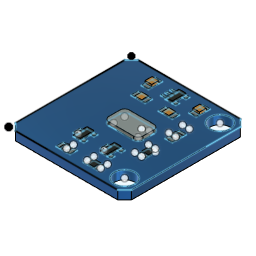
MPL3115A2 (Autodesk Fusion 360 design; units mm, degrees)
Autodesk Fusion 360 part; units mm, degrees
sketch "Esquisse1" plane through (0, 0, 0) normal (0, 0, 1) x (1, 0, 0)
  line L0 (1, 0) -> (16, 0)
  line L1 (17, 1) -> (17, 17)
  line L2 (16, 18) -> (1, 18)
  line L3 (0, 17) -> (0, 1)
  circle A0 centre (15, 16) radius 1.5
  circle A1 centre (15, 2) radius 1.5
  line L4 (10.8, 7.5) -> (7.2, 7.5)
  line L5 (6.5, 8.2) -> (6.5, 9.8)
  line L6 (7.2, 10.5) -> (10.8, 10.5)
  line L7 (11.5, 9.8) -> (11.5, 8.2)
  arc A2 (7.2, 10.5) -> (6.5, 9.8) centre (7.2, 9.8) ccw
  arc A3 (11.5, 9.8) -> (10.8, 10.5) centre (10.8, 9.8) ccw
  arc A4 (6.5, 8.2) -> (7.2, 7.5) centre (7.2, 8.2) ccw
  arc A5 (10.8, 7.5) -> (11.5, 8.2) centre (10.8, 8.2) ccw
  line L8 (14, 12) -> (13, 12)
  line L9 (13, 12) -> (13, 10)
  line L10 (13, 10) -> (14, 10)
  line L11 (14, 10) -> (14, 12)
  line L12 (14, 8) -> (13, 8)
  line L13 (13, 8) -> (13, 6)
  line L14 (13, 6) -> (14, 6)
  line L15 (14, 6) -> (14, 8)
  line L16 (12.5, 17) -> (11.5, 17)
  line L17 (11.5, 17) -> (11.5, 15)
  line L18 (11.5, 15) -> (12.5, 15)
  line L19 (12.5, 15) -> (12.5, 17)
  line L20 (12, 2) -> (10, 2)
  line L21 (10, 2) -> (10, 1)
  line L22 (10, 1) -> (12, 1)
  line L23 (12, 1) -> (12, 2)
  line L24 (8, 2) -> (6, 2)
  line L25 (6, 2) -> (6, 1)
  line L26 (6, 1) -> (8, 1)
  line L27 (8, 1) -> (8, 2)
  line L28 (10.97, 5.5) -> (10, 5.5)
  line L29 (10, 5.5) -> (10, 3.5)
  line L30 (10, 3.5) -> (10.97, 3.5)
  line L31 (10.97, 3.5) -> (10.97, 5.5)
  line L32 (7, 5.5) -> (6, 5.5)
  line L33 (6, 5.5) -> (6, 3.5)
  line L34 (6, 3.5) -> (7, 3.5)
  line L35 (7, 3.5) -> (7, 5.5)
  line L36 (7.5, 5) -> (7, 5)
  line L37 (7, 5) -> (7, 5.5)
  line L38 (7, 5.5) -> (7.5, 5.5)
  line L39 (7.5, 5.5) -> (7.5, 5)
  line L40 (7.5, 4) -> (7, 4)
  line L41 (7, 4) -> (7, 3.5)
  line L42 (7, 3.5) -> (7.5, 3.5)
  line L43 (7.5, 3.5) -> (7.5, 4)
  line L44 (6, 4.2) -> (6, 4.7949)
  line L45 (10, 4) -> (10, 4.7949)
  line L46 (10.97, 5.5) -> (11.5, 5.5)
  line L47 (11.5, 5.5) -> (11.5, 5)
  line L48 (11.5, 5) -> (10.97, 5)
  line L49 (10.97, 5) -> (10.97, 5.5)
  line L50 (10.97, 4) -> (11.5, 4)
  line L51 (11.5, 4) -> (11.5, 3.5)
  line L52 (11.5, 3.5) -> (10.97, 3.5)
  line L53 (10.97, 3.5) -> (10.97, 4)
  line L54 (10, 5.0146) -> (9.5, 5.0146)
  line L55 (9.5, 5.0146) -> (9.5, 4)
  line L56 (9.5, 4) -> (10, 4)
  line L57 (10, 4) -> (10, 5.0146)
  line L58 (6, 5.0146) -> (5.5, 5.0146)
  line L59 (5.5, 5.0146) -> (5.5, 4)
  line L60 (5.5, 4) -> (6, 4)
  line L61 (6, 4) -> (6, 5.0146)
  line L62 (9, 17) -> (8, 17)
  line L63 (8, 17) -> (8, 15)
  line L64 (8, 15) -> (9, 15)
  line L65 (9, 15) -> (9, 17)
  line L66 (9.5, 15.5) -> (9, 15.5)
  line L67 (9, 15.5) -> (9, 15)
  line L68 (9, 15) -> (9.5, 15)
  line L69 (9.5, 15) -> (9.5, 15.5)
  line L70 (9.5, 17) -> (9, 17)
  line L71 (9, 17) -> (9, 16.5)
  line L72 (9, 16.5) -> (9.5, 16.5)
  line L73 (9.5, 16.5) -> (9.5, 17)
  line L74 (8, 16.5) -> (7.2, 16.5)
  line L75 (7.2, 16.5) -> (7.2, 16.75)
  line L76 (7.2, 16.75) -> (8, 16.75)
  line L77 (8, 16.75) -> (8, 16.5)
  line L78 (8, 15.7969) -> (7.2, 15.7969)
  line L79 (7.2, 15.7969) -> (7.2, 16.0489)
  line L80 (7.2, 16.0489) -> (8, 16.0489)
  line L81 (8, 16.0489) -> (8, 15.7969)
  line L82 (8, 15.4) -> (7.2, 15.4)
  line L83 (7.2, 15.4) -> (7.2, 15.1433)
  line L84 (7.2, 15.1433) -> (8, 15.1433)
  line L85 (8, 15.1433) -> (8, 15.4)
  line L86 (5.5, 17) -> (4.5, 17)
  line L87 (4.5, 15) -> (5.5, 15)
  line L88 (4.5, 17) -> (4.5, 15)
  line L89 (5.5, 15) -> (5.5, 17)
  line L90 (11, 14) -> (9, 14)
  line L91 (9, 14) -> (9, 13)
  line L92 (9, 13) -> (11, 13)
  line L93 (11, 13) -> (11, 14)
  line L94 (7, 14) -> (5, 14)
  line L95 (5, 14) -> (5, 13)
  line L96 (5, 13) -> (7, 13)
  line L97 (7, 13) -> (7, 14)
  line L98 (5.5, 14) -> (5.5, 13)
  line L99 (6.5, 14) -> (6.5, 13)
  line L100 (9.5, 14) -> (9.5, 13)
  line L101 (10.5, 14) -> (10.5, 13)
  line L102 (4.5, 16.5273) -> (5.5, 16.5273)
  line L103 (4.5, 15.4891) -> (5.5, 15.4891)
  line L104 (11.5, 15.5) -> (12.5, 15.5)
  line L105 (11.5, 16.5273) -> (12.5, 16.5273)
  line L106 (6.5, 2) -> (6.5, 1)
  line L107 (7.5, 2) -> (7.5, 1)
  line L108 (10.5, 2) -> (10.5, 1)
  line L109 (11.5, 2) -> (11.5, 1)
  line L110 (13, 7.5) -> (14, 7.5)
  line L111 (13, 6.5) -> (14, 6.5)
  line L112 (13, 11.5) -> (14, 11.5)
  line L113 (14, 10.5) -> (13, 10.5)
  line L114 (16, 18) -> (17, 17)
  line L115 (16, 0) -> (17, 1)
  line L116 (0, 17) -> (1, 18)
  line L117 (0, 1) -> (1, 0)
  point P0 (0, 18)
  dimension "d2" = 18
  dimension "d3" = 3
  dimension "d4" = 3
  dimension "d11" = 0.7
  dimension "d12" = 0.7
  constraint horizontal L0
  constraint vertical L1
  constraint horizontal L2
  constraint vertical L3
  constraint perpendicular L3 L4
  constraint perpendicular L4 L5
  constraint perpendicular L5 L6
  constraint perpendicular L4 L7
  constraint tangent L5 A2
  constraint tangent L6 A2
  constraint tangent L6 A3
  constraint tangent L7 A3
  constraint tangent L4 A4
  constraint tangent L5 A4
  constraint equal A3 A4
  constraint tangent L4 A5
  constraint tangent L7 A5
  constraint equal A3 A5
  constraint coincident origin L0
  constraint coincident origin L3
  constraint coincident P0 L2
  constraint coincident P0 L3
  constraint horizontal L8
  constraint vertical L9
  constraint horizontal L10
  constraint vertical L11
  constraint horizontal L12
  constraint vertical L13
  constraint horizontal L14
  constraint vertical L15
  constraint horizontal L16
  constraint vertical L17
  constraint horizontal L18
  constraint vertical L19
  constraint horizontal L20
  constraint vertical L21
  constraint horizontal L22
  constraint vertical L23
  constraint horizontal L24
  constraint vertical L25
  constraint horizontal L26
  constraint vertical L27
  constraint horizontal L28
  constraint vertical L29
  constraint horizontal L30
  constraint vertical L31
  constraint horizontal L32
  constraint vertical L33
  constraint horizontal L34
  constraint vertical L35
  constraint horizontal L36
  constraint vertical L37
  constraint horizontal L38
  constraint vertical L39
  constraint horizontal L40
  constraint vertical L41
  constraint horizontal L42
  constraint vertical L43
  constraint vertical L44
  constraint coincident L33 L44.end
  constraint vertical L45
  constraint coincident L29 L45.end
  constraint horizontal L46
  constraint vertical L47
  constraint horizontal L48
  constraint vertical L49
  constraint horizontal L50
  constraint vertical L51
  constraint horizontal L52
  constraint vertical L53
  constraint coincident L31 L50.start
  constraint horizontal L54
  constraint vertical L55
  constraint horizontal L56
  constraint vertical L57
  constraint coincident L29 L54.start
  constraint horizontal L58
  constraint vertical L59
  constraint horizontal L60
  constraint vertical L61
  constraint coincident L33 L58.start
  constraint horizontal L62
  constraint vertical L63
  constraint horizontal L64
  constraint vertical L65
  constraint horizontal L66
  constraint vertical L67
  constraint horizontal L68
  constraint vertical L69
  constraint horizontal L70
  constraint vertical L71
  constraint horizontal L72
  constraint vertical L73
  constraint coincident L65 L71.end
  constraint horizontal L74
  constraint vertical L75
  constraint horizontal L76
  constraint vertical L77
  constraint coincident L63 L74.start
  constraint horizontal L78
  constraint vertical L79
  constraint horizontal L80
  constraint vertical L81
  constraint coincident L63 L78.start
  constraint horizontal L82
  constraint vertical L83
  constraint horizontal L84
  constraint vertical L85
  constraint coincident L63 L82.start
  constraint horizontal L86
  constraint vertical L88
  constraint horizontal L87
  constraint vertical L89
  constraint horizontal L90
  constraint vertical L91
  constraint horizontal L92
  constraint vertical L93
  constraint horizontal L94
  constraint vertical L95
  constraint horizontal L96
  constraint vertical L97
  constraint coincident L94 L98.start
  constraint coincident L96 L98.end
  constraint perpendicular L96 L98
  constraint coincident L94 L99.start
  constraint coincident L96 L99.end
  constraint perpendicular L96 L99
  constraint coincident L90 L100.start
  constraint coincident L92 L100.end
  constraint perpendicular L92 L100
  constraint coincident L90 L101.start
  constraint coincident L92 L101.end
  constraint perpendicular L92 L101
  constraint coincident L88 L102.start
  constraint coincident L89 L102.end
  constraint perpendicular L89 L102
  constraint coincident L88 L103.start
  constraint coincident L89 L103.end
  constraint perpendicular L89 L103
  constraint coincident L17 L104.start
  constraint coincident L19 L104.end
  constraint perpendicular L19 L104
  constraint coincident L17 L105.start
  constraint coincident L19 L105.end
  constraint perpendicular L19 L105
  constraint coincident L24 L106.start
  constraint coincident L26 L106.end
  constraint perpendicular L26 L106
  constraint coincident L24 L107.start
  constraint coincident L26 L107.end
  constraint perpendicular L26 L107
  constraint coincident L20 L108.start
  constraint coincident L22 L108.end
  constraint perpendicular L22 L108
  constraint coincident L20 L109.start
  constraint coincident L22 L109.end
  constraint perpendicular L22 L109
  constraint coincident L13 L110.start
  constraint perpendicular L13 L110
  constraint coincident L13 L111.start
  constraint coincident L15 L111.end
  constraint perpendicular L15 L111
  constraint coincident L9 L112.start
  constraint coincident L11 L112.end
  constraint perpendicular L11 L112
  constraint coincident L11 L113.start
  constraint coincident L9 L113.end
  constraint perpendicular L9 L113
  measures "d2" distance of origin P0
  measures "d3" diameter of A0
  measures "d4" diameter of A1
  measures "d11" radius of A2
  measures "d12" radius of A3
extrude "Extrusion1" add sketch "Esquisse1" against normal blind 1.27 contours L0 L1 L2 L3 L114 L115 L116 L117 | L4 L5 L6 L7 A2 A3 A4 A5 | L8 L9 L11 L112 | L9 L11 L112 L113 | L9 L10 L11 L113 | L12 L13 L15 L110 | L13 L15 L110 L111 | L13 L14 L15 L111 | L16 L17 L19 L105 | L17 L19 L104 L105 | L17 L18 L19 L104 | L20 L22 L23 L109 | L20 L22 L108 L109 | L20 L21 L22 L108 | L24 L26 L27 L107 | L24 L26 L106 L107 | L24 L25 L26 L106 | L28 L29 L30 L31 L45 L49 L53 L57 | L31 L46 L47 L48 L49 | L29 L45 L54 L55 L56 L57 | L31 L50 L51 L52 L53 | L32 L33 L34 L35 L37 L41 L44 L61 | L35 L36 L37 L38 L39 | L33 L44 L58 L59 L60 L61 | L35 L40 L41 L42 L43 | L62 L63 L64 L65 L67 L71 L77 L81 L85 | L65 L70 L71 L72 L73 | L63 L74 L75 L76 L77 | L65 L66 L67 L68 L69 | L63 L78 L79 L80 L81 | L63 L82 L83 L84 L85 | L86 L88 L89 L102 | L88 L89 L102 L103 | L87 L88 L89 L103 | L90 L92 L93 L101 | L90 L92 L100 L101 | L90 L91 L92 L100 | L94 L96 L97 L99 | L94 L96 L98 L99 | L94 L95 L96 L98 makes body 1
extrude "Extrusion2" add sketch "Esquisse1" along normal blind 0.5 separate body contours L4 L5 L6 L7 A2 A3 A4 A5 makes body 2
sketch "Esquisse2" plane through (0, 0, 0.5) normal (0, 0, 1) x (-1, 0, 0)
  arc A0 (-6.5, -8.2) -> (-7.2, -7.5) centre (-7.2, -8.2) ccw
  line L0 (-7.2, -7.5) -> (-10.8, -7.5)
  arc A1 (-10.8, -7.5) -> (-11.5, -8.2) centre (-10.8, -8.2) ccw
  line L1 (-11.5, -8.2) -> (-11.5, -9.8)
  arc A2 (-11.5, -9.8) -> (-10.8, -10.5) centre (-10.8, -9.8) ccw
  line L2 (-10.8, -10.5) -> (-7.2, -10.5)
  arc A3 (-7.2, -10.5) -> (-6.5, -9.8) centre (-7.2, -9.8) ccw
  line L3 (-6.5, -9.8) -> (-6.5, -8.2)
  circle A4 centre (-10.5, -9) radius 0.15
  line L4 (-7.5, -2) -> (-7.5, -1)
  line L5 (-10.5, -2) -> (-10.5, -1)
  line L6 (-12.5, -2) -> (-12.5, -1)
  line L7 (-13, -7.5) -> (-14, -7.5)
  line L8 (-13, -5.5) -> (-14, -5.5)
  line L9 (-13, -12.5) -> (-14, -12.5)
  line L10 (-13, -10.5) -> (-14, -10.5)
  dimension "d14" = 0.3
  constraint vertical L4
  constraint vertical L5
  constraint vertical L6
  constraint parallel L2 L7
  constraint horizontal L8
  constraint horizontal L9
  constraint horizontal L10
  measures "d14" diameter of A4
extrude "Extrusion3" cut sketch "Esquisse2" against normal blind 0.05 contours A4 bodies 2
extrude "Extrusion4" add sketch "Esquisse1" along normal blind 0.1 separate body contours L8 L9 L11 L112 | L9 L10 L11 L113 | L12 L13 L15 L110 | L13 L14 L15 L111 | L16 L17 L19 L105 | L17 L18 L19 L104 | L20 L22 L23 L109 | L20 L21 L22 L108 | L24 L26 L27 L107 | L24 L25 L26 L106 | L31 L46 L47 L48 L49 | L29 L45 L54 L55 L56 L57 | L31 L50 L51 L52 L53 | L35 L36 L37 L38 L39 | L33 L44 L58 L59 L60 L61 | L35 L40 L41 L42 L43 | L65 L70 L71 L72 L73 | L63 L74 L75 L76 L77 | L65 L66 L67 L68 L69 | L63 L78 L79 L80 L81 | L63 L82 L83 L84 L85 | L86 L88 L89 L102 | L87 L88 L89 L103 | L90 L92 L93 L101 | L90 L91 L92 L100 | L94 L96 L97 L99 | L94 L95 L96 L98 makes body 3 at (7.6667, 1.6667, 0) makes body 4 at (7.1667, 5.3333, 0) makes body 5 at (13.3333, 7.6667, 0) makes body 6 at (11.8333, 16.8424, 0) makes body 7 at (9.1667, 15.3333, 0) makes body 8 at (7.7333, 15.2288, 0) makes body 9 at (4.8333, 15.326, 0) makes body 10 at (6.6667, 13.6667, 0) makes body 11 at (9.1667, 16.8333, 0) makes body 12 at (11.8333, 15.3333, 0) makes body 13 at (13.3333, 6.1667, 0) makes body 14 at (11.3233, 3.8333, 0) makes body 15 at (6.1667, 1.6667, 0) makes body 16 at (10.1667, 1.6667, 0) makes body 17 at (7.1667, 3.8333, 0) makes body 18 at (11.3233, 5.1667, 0) makes body 19 at (13.3333, 11.8333, 0) makes body 20 at (9.1667, 13.6667, 0) makes body 21 at (7.4667, 15.8809, 0) makes body 22 at (4.8333, 16.8424, 0) makes body 23 at (5.3333, 13.3333, 0) makes body 24 at (7.4667, 16.5833, 0) makes body 25 at (10.6667, 13.6667, 0) makes body 26 at (13.3333, 10.3333, 0) makes body 27 at (9.6667, 4.6764, 0) makes body 28 at (5.6667, 4.3382, 0) makes body 29 at (11.6667, 1.6667, 0)
extrude "Extrusion5" add sketch "Esquisse1" along normal blind 0.2 separate body contours L9 L11 L112 L113 | L13 L15 L110 L111 | L20 L22 L108 L109 | L24 L26 L106 L107 | L90 L92 L100 L101 | L94 L96 L98 L99 makes body 30 at (6.8333, 1.6667, 0) makes body 31 at (6.1667, 13.6667, 0) makes body 32 at (10.8333, 1.6667, 0) makes body 33 at (13.3333, 11.1667, 0) makes body 34 at (9.8333, 13.6667, 0) makes body 35 at (13.3333, 7.1667, 0)
extrude "Extrusion6" add sketch "Esquisse1" along normal blind 0.3 separate body contours L28 L29 L30 L31 L45 L49 L53 L57 | L32 L33 L34 L35 L37 L41 L44 L61 | L62 L63 L64 L65 L67 L71 L77 L81 L85 makes body 36 at (6.3333, 4.8333, 0) makes body 37 at (10.3233, 4.8333, 0) makes body 38 at (8.3333, 16.3333, 0)
extrude "Extrusion7" add sketch "Esquisse1" along normal blind 0.4 separate body contours L17 L19 L104 L105 | L88 L89 L102 L103 makes body 39 at (4.8333, 16.1813, 0) makes body 40 at (11.8333, 16.1849, 0)
